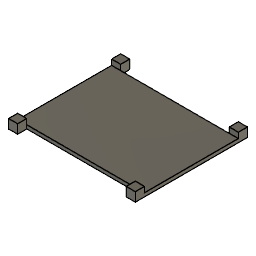
Case TOP(f3d) (Autodesk Fusion 360 design; units mm, degrees)
part number: 2026-08-19-01-06-16-783
Autodesk Fusion 360 part; units mm, degrees
sketch "Sketch1" plane through (0, 0, 0) normal (0, 0, 1) x (1, 0, 0)
  line L0 (34.65, 25.65) -> (-34.65, 25.65)
  line L1 (-34.65, 25.65) -> (-34.65, -25.65)
  line L2 (-34.65, -25.65) -> (34.65, -25.65)
  line L3 (34.65, -25.65) -> (34.65, 25.65)
  line L4 (34.65, 25.65) -> (-34.65, -25.65) construction
  line L5 (-34.65, 25.65) -> (34.65, -25.65) construction
  dimension "d1" = 69.3
  dimension "d2" = 51.3
  constraint horizontal L0
  constraint perpendicular L0 L1
  constraint parallel L0 L2
  constraint parallel L1 L3
  constraint coincident L4 origin
  constraint coincident L5 origin
  measures "d1" distance of L1.end L2.end
  measures "d2" distance of L0.end L1.end
extrude "Extrude1" add sketch "Sketch1" along normal blind 2
sketch "Sketch2" plane through (0, 0, 2) normal (0, 0, 1) x (-1, 0, 0)
  line L0 (-34.65, 25.65) -> (-34.65, -25.65)
  line L1 (-34.65, -25.65) -> (34.65, -25.65)
  line L2 (34.65, -25.65) -> (34.65, 25.65)
  line L3 (34.65, 25.65) -> (-34.65, 25.65)
  line L4 (34.65, -25.65) -> (29.65, -25.65)
  line L5 (29.65, -25.65) -> (29.65, -30.65)
  line L6 (29.65, -30.65) -> (34.65, -30.65)
  line L7 (34.65, -30.65) -> (34.65, -25.65)
  line L8 (-34.65, -25.65) -> (-29.65, -25.65)
  line L9 (-29.65, -25.65) -> (-29.65, -30.65)
  line L10 (-29.65, -30.65) -> (-34.65, -30.65)
  line L11 (-34.65, -30.65) -> (-34.65, -25.65)
  line L12 (34.65, 25.65) -> (29.65, 25.65)
  line L13 (29.65, 25.65) -> (29.65, 30.65)
  line L14 (29.65, 30.65) -> (34.65, 30.65)
  line L15 (34.65, 30.65) -> (34.65, 25.65)
  line L16 (-34.65, 25.65) -> (-29.65, 25.65)
  line L17 (-29.65, 25.65) -> (-29.65, 30.65)
  line L18 (-29.65, 30.65) -> (-34.65, 30.65)
  line L19 (-34.65, 30.65) -> (-34.65, 25.65)
  dimension "d5" = 5
  dimension "d6" = 5
  dimension "d7" = 5
  dimension "d8" = 5
  dimension "d9" = 5
  dimension "d10" = 5
  dimension "d11" = 5
  dimension "d12" = 5
  constraint horizontal L4
  constraint vertical L5
  constraint horizontal L6
  constraint vertical L7
  constraint coincident L1.end L2.start
  constraint horizontal L8
  constraint vertical L9
  constraint horizontal L10
  constraint vertical L11
  constraint coincident L0.end L1.start
  constraint horizontal L12
  constraint vertical L13
  constraint horizontal L14
  constraint vertical L15
  constraint coincident L2.end L3.start
  constraint horizontal L16
  constraint vertical L17
  constraint horizontal L18
  constraint vertical L19
  constraint coincident L0.start L3.end
  measures "d5" distance of L1.end L4.end
  measures "d6" distance of L1.end L6.end
  measures "d7" distance of L0.end L8.end
  measures "d8" distance of L0.end L10.end
  measures "d9" distance of L2.end L12.end
  measures "d10" distance of L2.end L14.end
  measures "d11" distance of L0.start L16.end
  measures "d12" distance of L0.start L18.end
extrude "Extrude2" add sketch "Sketch2" along normal blind 5 from surface at -2 contours L3 L16 L17 L18 L19 | L1 L8 L9 L10 L11 | L3 L12 L13 L14 L15 | L1 L4 L5 L6 L7
sketch "Sketch3" plane through (0, 0, 0) normal (0, 0, -1) x (1, 0, 0)
  line L0 (34.65, -30.65) -> (34.65, 30.65)
  line L1 (34.65, 30.65) -> (29.65, 30.65)
  line L2 (29.65, 30.65) -> (29.65, 25.65)
  line L3 (29.65, 25.65) -> (-29.65, 25.65)
  line L4 (-29.65, 25.65) -> (-29.65, 30.65)
  line L5 (-29.65, 30.65) -> (-34.65, 30.65)
  line L6 (-34.65, 30.65) -> (-34.65, -30.65)
  line L7 (-34.65, -30.65) -> (-29.65, -30.65)
  line L8 (-29.65, -30.65) -> (-29.65, -25.65)
  line L9 (-29.65, -25.65) -> (29.65, -25.65)
  line L10 (29.65, -25.65) -> (29.65, -30.65)
  line L11 (29.65, -30.65) -> (34.65, -30.65)
  circle A0 centre (-32.15, 28.15) radius 1.6
  circle A1 centre (32.15, 28.15) radius 1.6
  circle A2 centre (32.15, -28.15) radius 1.6
  circle A3 centre (-32.15, -28.15) radius 1.6
  dimension "d16" = 3.2
  dimension "d17" = 3.2
  dimension "d18" = 3.2
  dimension "d19" = 3.2
  dimension "d20" = 2.5
  dimension "d21" = 2.5
  dimension "d22" = 2.5
  dimension "d23" = 2.5
  dimension "d24" = 2.5
  dimension "d25" = 2.5
  dimension "d26" = 2.5
  dimension "d27" = 2.5
  measures "d16" diameter of A0
  measures "d17" diameter of A1
  measures "d18" diameter of A2
  measures "d19" diameter of A3
  measures "d20" distance of L6 A0.centre
  measures "d21" distance of L5 A0.centre
  measures "d22" distance of L1 A1.centre
  measures "d23" distance of L0 A1.centre
  measures "d24" distance of L0 A2.centre
  measures "d25" distance of L11 A2.centre
  measures "d26" distance of L8 A3.centre
  measures "d27" distance of L7 A3.centre
extrude "Extrude3" cut sketch "Sketch3" against normal blind 3.1 contours A0 | A1 | A2 | A3
